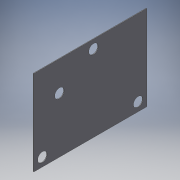
# Autodesk Inventor part: waterjet wall
Saved by Autodesk Inventor 2018 (Build 220112000, 112)
## iProperties
Created: 2020-01-24
Part Number: waterjet wall
Material: Generic
Document SubType Name: Modeling
Designer: s-2513225
Density: 1 g/cm^3
Appearance: Default
Author: s-2513225
Autodesk Inventor part; units mm, degrees
ref_plane "YZ Plane" through (0, 0, 0) normal (1, 0, 0) x (0, 1, 0)
ref_plane "XZ Plane" through (0, 0, 0) normal (0, 1, 0) x (-1, 0, 0)
ref_plane "XY Plane" through (0, 0, 0) normal (0, 0, 1) x (1, 0, 0)
sketch "Sketch1" plane through (0, 0, 0) normal (1, 0, 0) x (0, 1, 0)
  circle A0 centre (0, 0) radius 88.9 construction
  line L0 (-88.9, 0) -> (88.9, 0) construction
  line L1 (-88.9, -52.1993) -> (-88.9, 151.0007)
  line L2 (88.9, 0) -> (117.4115, 0) construction
  line L3 (-88.9, -128.3993) -> (-88.9, -52.1993)
  line L4 (165.1, -128.3993) -> (165.1, 151.0007)
  line L5 (165.1, 151.0007) -> (-88.9, 151.0007)
  line L6 (-88.9, 151.0007) -> (-63.5, 151.0007) construction
  line L7 (-63.5, 151.0007) -> (-63.5, 125.6007) construction
  circle A1 centre (-63.5, 125.6007) radius 14.2875
  line L8 (-63.5, 125.6007) -> (-63.5, -26.7993) construction
  line L9 (-63.5, -26.7993) -> (139.7, -26.7993) construction
  circle A2 centre (139.7, -26.7993) radius 14.2875
  line L10 (-63.5, 125.6007) -> (76.2, 125.6007) construction
  line L11 (76.2, 125.6007) -> (76.2, 74.8007) construction
  circle A3 centre (76.2, 74.8007) radius 14.2875
  line L12 (-88.9, -128.3993) -> (-88.9, -179.1993)
  line L13 (-88.9, -179.1993) -> (-88.9, -185.5493)
  line L14 (-88.9, -185.5493) -> (165.1, -185.5493)
  line L15 (165.1, -185.5493) -> (165.1, -128.3993)
  dimension "d0" = 177.8
  dimension "d1" = 203.2
  dimension "d2" = 28.5115
  dimension "d4" = 76.2
  dimension "d5" = 279.4
  dimension "d8" = 25.4
  dimension "d9" = 25.4
  dimension "d10" = 28.575
  dimension "d11" = 152.4
  dimension "d12" = 203.2
  dimension "d13" = 28.575
  dimension "d14" = 139.7
  dimension "d15" = 50.8
  dimension "d16" = 28.575
  dimension "d19" = 50.8
  dimension "d21" = 6.35
  dimension "d22" = 254
  constraints: 32 end point, 5 perpendicular, 4 centre point, 4 coincident, 4 vertical, 3 horizontal, 2 point on circle, 2 point on line, 1 parallel
  measures "d0" diameter of A0
  measures "d1" distance of L1.start L1.end
  measures "d2" distance of L0.end L2.end
  measures "d4" distance of L3.start L1.start
  measures "d5" distance of L4.start L4.end
  measures "d8" distance of L5.end L6.end
  measures "d9" distance of L6.end L7.end
  measures "d10" diameter of A1
  measures "d11" distance of L8.start L8.end
  measures "d12" distance of L8.end L9.end
  measures "d13" diameter of A2
  measures "d14" distance of L8.start L10.end
  measures "d15" distance of L10.end L11.end
  measures "d16" diameter of A3
  measures "d19" distance of L3.start L12.end
  measures "d21" distance of L12.end L13.end
  measures "d22" distance of L13.end L14.end
extrude "Extrusion2" add sketch "Sketch1" along normal blind 1.778
sketch "Sketch2" plane through (1.778, 0, 0) normal (1, 0, 0) x (0, 0, -1)
  line L0 (185.5493, -88.9) -> (185.5493, 165.1) construction
  line L1 (185.5493, -88.9) -> (160.1493, -88.9) construction
  line L2 (-151.0007, -88.9) -> (185.5493, -88.9) construction
  line L3 (160.1493, -88.9) -> (160.1493, -63.5) construction
  line L4 (160.1493, -63.5) -> (185.5493, -63.5) construction
  circle A0 centre (160.1493, -63.5) radius 14.2875
  point P0 (0, 0)
  dimension "d23" = 25.4
  dimension "d24" = 25.4
  dimension "d25" = 28.575
  constraints: 6 end point, 2 perpendicular, 1 centre point, 1 coincident, 1 point on line
  measures "d23" distance of L0.start L1.end
  measures "d24" distance of L1.end L3.end
  measures "d25" diameter of A0
extrude "Extrusion3" cut sketch "Sketch2" against normal blind 1.778
body "Solid2"
